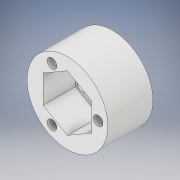
# Autodesk Inventor part: AA050
Saved by Autodesk Inventor 2017 SP1 (Build 210196100, 196)
## iProperties
Created: 2018-02-16
Part Number: AA050
Material: ABS Plastic
Document SubType Name: Modeling
Designer: Zach
Density: 1.06 g/cm^3
Appearance: CR White
Author: Zach
Autodesk Inventor part; units mm, degrees
ref_plane "YZ Plane" through (0, 0, 0) normal (1, 0, 0) x (0, 1, 0)
ref_plane "XZ Plane" through (0, 0, 0) normal (0, 1, 0) x (-1, 0, 0)
ref_plane "XY Plane" through (0, 0, 0) normal (0, 0, 1) x (1, 0, 0)
sketch "Sketch1" plane through (0, 0, 0) normal (0, 0, 1) x (1, 0, 0)
  circle A0 centre (0, 0) radius 12.5
  circle A1 centre (0, 0) radius 2.5
  circle A2 centre (9.525, 0) radius 1.5
  circle A3 centre (-4.7625, 8.2489) radius 1.5
  circle A4 centre (-4.7625, -8.2489) radius 1.5
  circle A5 centre (5.4993, 3.175) radius 1.5
  line L0 (0, 0) -> (5.4993, 3.175) construction
  line L1 (0, 0) -> (17.6195, 0) construction
  circle A6 centre (-5.4993, -3.175) radius 1.5
  dimension "d0" = 25
  dimension "d1" = 5
  dimension "d2" = 3
  dimension "d3" = 9.525
  dimension "d6" = 360
  dimension "d8" = 3
  dimension "d10" = 6.35
  dimension "d11" = 30
  dimension "d14" = 360
  constraints: 7 centre point, 4 end point, 2 coincident, 1 horizontal, 1 horizontal alignment, 12 other
  measures "d0" diameter of A0
  measures "d1" diameter of A1
  measures "d2" diameter of A2
  measures "d3" distance of A2.centre point (0, 0)
  measures "d8" diameter of A5
  measures "d10" distance of L0.start L0.end
  measures "d11" angle of L0 L1
extrude "Extrusion1" add sketch "Sketch1" along normal blind 14
sketch "Sketch2" plane through (0, 0, 14) normal (0, 0, 1) x (1, 0, 0)
  circle A0 centre (0, 0) radius 2.5 construction
  line L0 (0, 8.6603) -> (7.5, 4.3301)
  line L1 (7.5, 4.3301) -> (7.5, -4.3301)
  line L2 (7.5, -4.3301) -> (0, -8.6603)
  line L3 (0, -8.6603) -> (-7.5, -4.3301)
  line L4 (-7.5, -4.3301) -> (-7.5, 4.3301)
  line L5 (-7.5, 4.3301) -> (0, 8.6603)
  circle A1 centre (9.525, 0) radius 1.5 construction
  line L6 (0, 0) -> (9.525, 0) construction
  point P0 (7.5, 0)
  dimension "d18" = 15
  constraints: 14 end point, 1 coincident, 1 horizontal, 1 midpoint, 1 point on line, 13 other
  measures "d18" distance between parallel lines of L2 L5
extrude "Extrusion2" cut sketch "Sketch2" against normal blind 10
body "Solid1"
